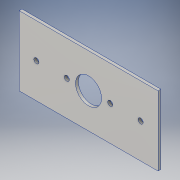
# Autodesk Inventor part: GearboxPlate
Saved by Autodesk Inventor 2016 (Build 200138000, 138)
## iProperties
Created: 2017-01-19
Part Number: GearboxPlate
Material: Aluminum 6061
Document SubType Name: Modeling
Designer: Kyle
Density: 2.7 g/cm^3
Appearance: Aluminum - Flat
Author: Kyle
Autodesk Inventor part; units mm, degrees
ref_plane "YZ Plane" through (0, 0, 0) normal (1, 0, 0) x (0, 1, 0)
ref_plane "XZ Plane" through (0, 0, 0) normal (0, 1, 0) x (-1, 0, 0)
ref_plane "XY Plane" through (0, 0, 0) normal (0, 0, 1) x (1, 0, 0)
sketch "Sketch1" plane through (0, 0, 0) normal (0, 0, 1) x (1, 0, 0)
  line L0 (0, 0) -> (152.4, 0)
  line L1 (152.4, 0) -> (152.4, 76.2)
  line L2 (152.4, 76.2) -> (0, 76.2)
  line L3 (0, 76.2) -> (0, 0)
  dimension "d0" = 152.4
  dimension "d1" = 76.2
  constraints: 8 end point, 2 parallel, 1 horizontal, 1 perpendicular
  measures "d0" distance of L2.end L1.end
  measures "d1" distance of L1.end L0.end
extrude "Extrusion1" add sketch "Sketch1" along normal blind 3.175
sketch "Sketch2" plane through (0, 0, 3.175) normal (0, 0, 1) x (1, 0, 0)
  circle A0 centre (76.2, 38.1) radius 14.2875
  line L0 (152.4, 76.2) -> (0, 76.2) projected
  line L1 (0, 76.2) -> (0, 0) projected
  circle A1 centre (52.3875, 38.1) radius 2.8067
  circle A2 centre (100.0125, 38.1) radius 2.8067
  circle A3 centre (19.05, 38.1) radius 2.8067
  circle A4 centre (133.35, 38.1) radius 2.8067
  dimension "d4" = 28.575
  dimension "d5" = 38.1
  dimension "d6" = 76.2
  dimension "d8" = 5.6134
  dimension "d9" = 5.6134
  dimension "d11" = 5.6134
  dimension "d12" = 5.6134
  constraints: 5 centre point
  measures "d4" diameter of A0
  measures "d5" distance from line of L0 A0.centre
  measures "d6" distance from line of L1 A0.centre
  measures "d8" diameter of A1
  measures "d9" diameter of A2
  measures "d11" diameter of A3
  measures "d12" diameter of A4
extrude "Extrusion2" cut sketch "Sketch2" against normal blind 3.175
body "Solid1"
